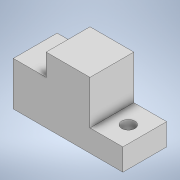
# Autodesk Inventor part: 1.3
Saved by Autodesk Inventor 2022 (Build 260153000, 153)
## iProperties
Created: 2023-04-17
Part Number: 1.3
Material: Genérico
Document SubType Name: Modeling
Designer: jpjoa
Density: 1 g/cm^3
Appearance: Padrão
Author: jpjoa
Autodesk Inventor part; units mm, degrees
ref_plane "YZ Plane" through (0, 0, 0) normal (1, 0, 0) x (0, 1, 0)
ref_plane "XZ Plane" through (0, 0, 0) normal (0, 1, 0) x (-1, 0, 0)
ref_plane "XY Plane" through (0, 0, 0) normal (0, 0, 1) x (1, 0, 0)
sketch "Esboço1" plane through (0, 0, 0) normal (0, 0, 1) x (1, 0, 0)
  line L0 (0, 0) -> (50, 0)
  line L1 (0, 0) -> (0, 20)
  line L2 (0, 20) -> (15, 20)
  line L3 (15, 20) -> (15, 30)
  line L4 (15, 30) -> (35, 30)
  line L5 (35, 30) -> (35, 10)
  line L6 (35, 10) -> (50, 10)
  line L7 (50, 10) -> (50, 0)
  dimension "d0" = 50
  dimension "d1" = 20
  dimension "d2" = 15
  dimension "d3" = 10
  dimension "d4" = 20
  dimension "d5" = 20
  dimension "d6" = 15
  constraints: 16 end point, 4 perpendicular, 2 horizontal, 1 vertical
  measures "d0" distance of L0.start L0.end
  measures "d1" distance of L0.start L1.end
  measures "d2" distance of L1.end L2.end
  measures "d3" distance of L2.end L3.end
  measures "d4" distance of L3.end L4.end
  measures "d5" distance of L4.end L5.end
  measures "d6" distance of L5.end L6.end
extrude "Extrusão1" add sketch "Esboço1" along normal blind 20
sketch "Esboço2" plane through (35, 10, 0) normal (0, 1, 0) x (1, 0, 0)
  circle A0 centre (7.5, -10) radius 3
  line L0 (15, 0) -> (15, -20) projected
  line L1 (15, -20) -> (0, -20) projected
  point P0 (-35, 0)
  dimension "d9" = 6
  dimension "d10" = 7.5
  dimension "d11" = 10
  constraints: 1 centre point
  measures "d9" diameter of A0
  measures "d10" distance from line of L0 A0.centre
  measures "d11" distance from line of L1 A0.centre
extrude "Extrusão2" cut sketch "Esboço2" against normal through all
